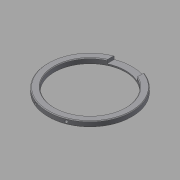
# Autodesk Inventor part: KE-SP-02-P1
Saved by Autodesk Inventor 2018 (Build 220112000, 112)
## iProperties
Created: 2015-08-04
Part Number: KE-SP-02-P1
Material: 一般
Document SubType Name: Modeling
Designer: ERIC
Density: 1 g/cm^3
Appearance: 預設
Author: ERIC
Autodesk Inventor part; units mm, degrees
sketch "草圖1" plane through (0, 0, 0) normal (0, 0, 1) x (1, 0, 0)
  circle A0 centre (0, 0) radius 30.85
  circle A1 centre (0, 0) radius 25.95
  dimension "d0" = 61.7
  dimension "d3" = 51.9
  constraints: 2 centre point, 2 coincident
  measures "d0" diameter of A0
  measures "d3" diameter of A1
extrude "擠出1" add sketch "草圖1" along normal blind 4
sketch "草圖2" plane through (0, 0, 4) normal (0, 0, 1) x (1, 0, 0)
  circle A0 centre (0, 0) radius 25.95 projected
  circle A1 centre (0, 0) radius 30.85 projected
  line L0 (0, 0) -> (0, 30.85)
  line L1 (11, 28.8223) -> (11, 23.5032)
  line L2 (-11, 28.8223) -> (-11, 23.5032)
  dimension "d6" = 22
  constraints: 6 end point, 5 point on circle, 2 parallel, 1 vertical, 1 other
  measures "d6" distance between parallel lines of L1 L2
extrude "擠出2" cut sketch "草圖2" against normal blind 2.5 contours A0 L0 A1 L1 | L2 A1 L0 A0
ref_plane "工作平面1" through (0, 0, 2) normal (0, 0, 1) x (1, 0, 0)
sketch "草圖3" plane through (0, 0, 2) normal (0, 0, 1) x (1, 0, 0)
  line L0 (0, 0) -> (0, -42.4806)
  line L1 (0, 0) -> (-11.25, -28.7256)
  line L2 (0, 0) -> (11.25, -28.7256)
  arc A0 (-11, 28.8223) -> (11, 28.8223) centre (0, 0) ccw projected
  line L3 (-11.25, -28.7256) -> (11.25, -28.7256)
  dimension "d9" = 22.5
  constraints: 8 end point, 2 point on circle, 1 perpendicular, 1 vertical, 1 other
  measures "d9" distance of L1.end L2.end
ref_plane "工作平面2" through (11.25, -28.7256, 2) normal (0.3647, -0.9311, 0) x (0.9311, 0.3647, 0)
ref_plane "工作平面3" through (-11.25, -28.7256, 2) normal (-0.3647, -0.9311, 0) x (0.9311, -0.3647, 0)
sketch "草圖4" plane through (11.25, -28.7256, 2) normal (0.3647, -0.9311, 0) x (0.9311, 0.3647, 0)
  point P0 (0, -2)
  point P1 (0, 0)
hole "孔1" at (11.25, -28.7256, 2) direction (-0.3647, 0.9311, 0) diameter 2 depth 2.5 tip angle 118
sketch "草圖5" plane through (-11.25, -28.7256, 2) normal (-0.3647, -0.9311, 0) x (0.9311, -0.3647, 0)
  point P0 (0, -2)
  point P1 (0, 0)
hole "孔2" at (-11.25, -28.7256, 2) direction (0.3647, 0.9311, 0) diameter 2 depth 2.5 tip angle 118
chamfer "倒角1" distance 0.5 angle 45 6 edges at (-13.9275, -21.8958, 4) (21.8958, 13.9275, 4) (-25.95, 0, 0) (-17.4982, -25.4074, 4) (25.4074, 17.4982, 4) (-30.85, 0, 0)
